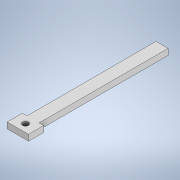
# Autodesk Inventor part: seddd
Saved by Autodesk Inventor 2020 (Build 240168000, 168)
## iProperties
Created: 2020-03-05
Part Number: seddd
Material: Generic
Document SubType Name: Modeling
Designer: Aryan
Density: 1 g/cm^3
Appearance: Default
Author: Aryan
Autodesk Inventor part; units mm, degrees
ref_plane "YZ Plane" through (0, 0, 0) normal (1, 0, 0) x (0, 1, 0)
ref_plane "XZ Plane" through (0, 0, 0) normal (0, 1, 0) x (-1, 0, 0)
ref_plane "XY Plane" through (0, 0, 0) normal (0, 0, 1) x (1, 0, 0)
sketch "Sketch1" plane through (0, 0, 0) normal (0, 1, 0) x (-1, 0, 0)
  line L0 (0, 0) -> (8, 0)
  line L1 (8, 0) -> (8, 85)
  line L2 (8, 85) -> (0, 85)
  line L3 (0, 85) -> (0, 0)
  dimension "d0" = 8
  dimension "d1" = 85
  constraints: 8 end point, 2 parallel, 1 horizontal, 1 perpendicular
  measures "d0" distance of L2.end L1.end
  measures "d1" distance of L1.end L0.end
extrude "Extrusion1" add sketch "Sketch1" along normal blind 4
sketch "Sketch2" plane through (0, 4, 0) normal (0, 1, 0) x (1, 0, 0)
  line L0 (-8, -85) -> (0, -85) projected
  line L1 (-4, -85) -> (-11, -85)
  line L2 (-11, -85) -> (-11, -95)
  line L3 (-11, -95) -> (-4, -95)
  line L4 (-4, -95) -> (-4, -85)
  point P0 (0, 0)
  dimension "d4" = 7
  dimension "d5" = 10
  constraints: 8 end point, 2 parallel, 1 horizontal, 1 midpoint, 1 perpendicular
  measures "d4" distance of L3.end L2.end
  measures "d5" distance of L2.end L1.end
extrude "Extrusion2" add sketch "Sketch2" against normal blind 4
sketch "Sketch3" plane through (0, 4, 0) normal (0, 1, 0) x (1, 0, 0)
  line L0 (-4, -85) -> (-4, -95) projected
  line L1 (-4, -85) -> (3, -85)
  line L2 (3, -85) -> (3, -95)
  line L3 (3, -95) -> (-4, -95)
  line L4 (-4, -95) -> (-4, -85)
  point P0 (0, 0)
  dimension "d8" = 7
  dimension "d9" = 10
  constraints: 8 end point, 2 parallel, 1 horizontal, 1 perpendicular
  measures "d8" distance of L2.end L3.end
  measures "d9" distance of L1.end L2.end
extrude "Extrusion3" add sketch "Sketch3" against normal blind 4
sketch "Sketch5" plane through (0, 4, 0) normal (0, 1, 0) x (1, 0, 0)
  line L0 (-11, -95) -> (-11, -85) projected
  line L1 (-11, -95) -> (-4, -95)
  line L2 (-4, -95) -> (-4, -90)
  line L3 (-4, -90) -> (-11, -90)
  line L4 (-11, -90) -> (-11, -95)
  circle A0 centre (-4, -90) radius 2
  point P0 (0, 0)
  dimension "d14" = 7
  dimension "d15" = 5
  dimension "d16" = 4
  constraints: 8 end point, 2 parallel, 1 centre point, 1 coincident, 1 horizontal, 1 perpendicular
  measures "d14" distance of L3.end L2.end
  measures "d15" distance of L2.end L1.end
  measures "d16" diameter of A0
extrude "Extrusion4" cut sketch "Sketch5" against normal blind 4 contours A0 L2 L3 | L3 L2 A0
body "Solid1"
